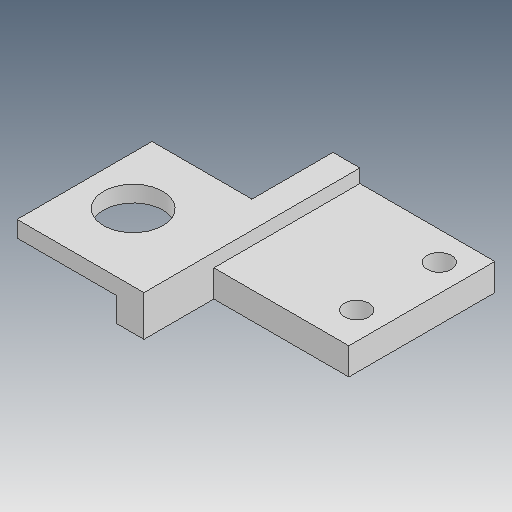
# Autodesk Inventor part: imu2_mount
Saved by Autodesk Inventor 2025.2 (Build 292293000, 293)
## iProperties
Created: 2025-02-23
Part Number: imu2_mount
Material: Generic
Document SubType Name: Modeling
Designer: email
Density: 1 g/cm^3
Appearance: Default
Author: email
Autodesk Inventor part; units mm, degrees
ref_plane "YZ Plane" through (0, 0, 0) normal (1, 0, 0) x (0, 1, 0)
ref_plane "XZ Plane" through (0, 0, 0) normal (0, 1, 0) x (-1, 0, 0)
ref_plane "XY Plane" through (0, 0, 0) normal (0, 0, 1) x (1, 0, 0)
sketch "Sketch1" plane through (0, 0, 0) normal (0, 1, 0) x (-1, 0, 0)
  line L0 (10, 7.5) -> (10, -7.5)
  circle A0 centre (0, 0) radius 5.25
  circle A1 centre (-15.9216, -7.65) radius 2.25
  circle A2 centre (-15.8711, 7.6499) radius 2.25
  line L1 (10, 0) -> (-25.8686, 0) construction
  line L2 (10, 7.5) -> (-10.3711, 7.5)
  line L3 (-10.3711, 7.5) -> (-10.3711, 15.9691)
  line L4 (-10.3711, 15.9691) -> (-21.3711, 15.9691)
  line L5 (-21.3711, 15.9691) -> (-21.3711, -15)
  line L6 (-21.3711, -15) -> (-10.3711, -15)
  line L7 (-10.3711, -15) -> (-10.3711, -7.5)
  line L8 (-10.3711, -7.5) -> (10, -7.5)
  circle A3 centre (-15.9216, -7.65) radius 5
  circle A4 centre (-15.8711, 7.6499) radius 4.9375
  point P0 (-7.9343, 0)
  dimension "d0" = 10.5
  dimension "d2" = 10
  dimension "d3" = 15.3
  dimension "d4" = 7.65
  dimension "d5" = 4.5
  dimension "d6" = 15
  dimension "d7" = 15
  dimension "d8" = 11
  dimension "d9" = 5.5
  dimension "d10" = 10
  constraints: 18 end point, 5 centre point, 5 perpendicular, 3 coincident, 2 midpoint, 2 point on line, 1 equal radius, 1 horizontal, 1 horizontal alignment
  measures "d0" diameter of A0
  measures "d2" distance of point (0, 0) L1.start
  measures "d3" distance of A2.centre A1.centre
  measures "d4" distance from line of L1 A1.centre
  measures "d5" diameter of A1
  measures "d6" distance between parallel lines of L2 L8
  measures "d7" distance from line of point (-7.934, 0) L6
  measures "d8" distance between parallel lines of L5 L3
  measures "d9" distance from line of L3 A2.centre
  measures "d10" diameter of A3
extrude "Extrusion1" [suppressed]
sketch "Sketch2" plane through (0, 0, 0) normal (0, 0, 1) x (1, 0, 0)
  line L0 (0, 0) -> (0, 3)
  line L1 (0, 3) -> (23.5, 3)
  line L2 (23.5, 3) -> (23.5, 0.5)
  line L3 (23.5, 0.5) -> (48.5, 0.5)
  line L4 (48.5, 0.5) -> (48.5, -4.5)
  line L5 (48.5, -4.5) -> (18.5, -4.5)
  line L6 (18.5, -4.5) -> (18.5, 0)
  line L7 (18.5, 0) -> (0, 0)
  line L8 (18.5, 0) -> (18.5, 3)
  point P0 (0, 1.5)
  dimension "d13" = 3
  dimension "d14" = 5
  dimension "d15" = 25
  dimension "d16" = 23.5
  dimension "d28" = 4.5
  dimension "d29" = 5
  constraints: 18 end point, 6 perpendicular, 2 vertical, 1 midpoint, 1 parallel, 1 point on line
  measures "d13" distance between parallel lines of L7 L1
  measures "d14" distance between parallel lines of L2 L6
  measures "d15" distance of L2.end L3.end
  measures "d16" distance from line of point (0, 1.5) L2
  measures "d28" distance between parallel lines of L5 L7
  measures "d29" distance between parallel lines of L5 L3
extrude "Extrusion2" add sketch "Sketch2" against normal blind 25
sketch "Sketch3" plane through (0, 3, 0) normal (0, 1, 0) x (-1, 0, 0)
  circle A0 centre (-9, -12.5) radius 5.5
  line L0 (0, 0) -> (0, -25) projected
  line L1 (-23.5, 0) -> (0, 0) projected
  point P0 (0, -12.5)
  point P1 (0, -12.5)
  dimension "d19" = 11
  dimension "d26" = 9
  dimension "d27" = 12.5
  constraints: 2 midpoint, 1 centre point
  measures "d19" diameter of A0
  measures "d26" distance of point (0, -12.5) A0.centre
  measures "d27" distance from line of L1 A0.centre
extrude "Extrusion3" cut sketch "Sketch3" against normal blind 25
extrude "Extrusion4" add sketch "Sketch2" against normal blind 40 contours L8 L1 L2 L3 L4 L5 L6
sketch "Sketch4" plane through (23.5, 0.5, 0) normal (0, 1, 0) x (1, 0, 0)
  circle A0 centre (20, 34.7005) radius 2.25
  circle A1 centre (20, 19.4005) radius 2.25
  line L0 (0, 0) -> (0, 40) projected
  point P0 (-23.5, 0)
  dimension "d32" = 4.5
  dimension "d33" = 15.3
  dimension "d36" = 20
  constraints: 2 centre point, 1 equal radius, 1 vertical alignment
  measures "d32" diameter of A0
  measures "d33" distance of A0.centre A1.centre
  measures "d36" distance from line of L0 A0.centre
extrude "Extrusion5" cut sketch "Sketch4" against normal up to surface (5 mm away)
sketch "Sketch5" plane through (23.5, 0.5, 0) normal (0, 1, 0) x (1, 0, 0)
  line L0 (25, 0) -> (0, 0) projected
  line L1 (0, 0) -> (0, 40) projected
  line L2 (25, 0) -> (0, 0)
  line L3 (0, 0) -> (0, 12.946)
  line L4 (0, 12.946) -> (25, 12.946)
  line L5 (25, 12.946) -> (25, 0)
  point P0 (-23.5, 0)
  constraints: 8 end point, 2 parallel, 1 horizontal, 1 perpendicular, 1 point on line
extrude "Extrusion6" cut sketch "Sketch5" against normal blind 10
equation "\"d4\" = 0.5 * d3"
body "Solid1"
